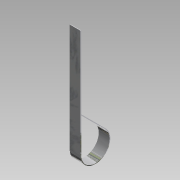
# Autodesk Inventor part: スタビライザ
Saved by Autodesk Inventor 2017 (Build 210142000, 142)
## iProperties
Part Number: スタビライザ
Material: アルミニウム
Document SubType Name: Modeling
Designer: HISAAKI
Density: 2.7 g/cm^3
Appearance: サテン
Author: HISAAKI
Autodesk Inventor part; units mm, degrees
ref_plane "YZ Plane" through (0, 0, 0) normal (1, 0, 0) x (0, 1, 0)
ref_plane "XZ Plane" through (0, 0, 0) normal (0, 1, 0) x (-1, 0, 0)
ref_plane "XY Plane" through (0, 0, 0) normal (0, 0, 1) x (1, 0, 0)
sketch "スケッチ3" plane through (0, 0, 0) normal (1, 0, 0) x (0, 1, 0)
  line L0 (0, 0) -> (0, -150)
  line L1 (0, 0) -> (0, -100)
  arc A0 (0, -150) -> (35.3553, -135.3553) centre (20.7107, -150) ccw
  line L2 (0, -150) -> (20.7107, -150) construction
  line L3 (35.3553, -135.3553) -> (20.7107, -150) construction
  line L4 (35.3553, -135.3553) -> (0, -100)
  line L5 (0, 0) -> (1, 0)
  arc A1 (1, -150) -> (34.6482, -136.0624) centre (20.7107, -150) ccw
  line L6 (34.6482, -136.0624) -> (1, -102.4142)
  line L7 (1, -150) -> (1, -102.4142)
  dimension "d13" = 150
  dimension "d14" = 100
  dimension "d16" = 135
  dimension "d17" = 1
  constraints: 16 end point, 4 point on circle, 3 point on line, 2 centre point, 2 tangent, 1 coincident, 1 horizontal, 1 parallel, 1 perpendicular, 1 vertical
  measures "d13" distance of L0.start L0.end
  measures "d14" distance of L0.start L1.end
  measures "d16" angle of L3 L2
  measures "d17" distance of L0.start L5.end
extrude "押し出し3" add sketch "スケッチ3" along normal blind 15
sketch "スケッチ4" plane through (0, 0, 0) normal (-1, 0, 0) x (0, 0, 1)
  line L0 (-100, 0) -> (-150, 0) projected
  line L1 (-100, 0) -> (0, 0)
  line L2 (0, 0) -> (0, 1)
  line L3 (0, 1) -> (-101, 1)
  line L4 (-135.3553, 35.3553) -> (-100, 0) projected
  line L5 (-101, 1) -> (-100, 0)
  dimension "d20" = 1
  constraints: 8 end point, 2 perpendicular, 1 collinear, 1 horizontal, 1 point on line
  measures "d20" distance of L1.end L2.end
extrude "押し出し4" add sketch "スケッチ4" against normal blind 15
sketch "スケッチ5" plane through (15, 0, 0) normal (1, 0, 0) x (0, 0, -1)
  line L0 (0, 0) -> (150, 0) projected
  line L1 (0, 0) -> (-10, 0)
  line L2 (-10, 0) -> (-10, 1)
  line L3 (-10, 1) -> (0, 1)
  line L4 (0, 1) -> (0, 0)
  dimension "d23" = 10
  dimension "d24" = 1
  constraints: 8 end point, 3 perpendicular, 1 horizontal
  measures "d23" distance of L0.start L1.end
  measures "d24" distance of L1.end L2.end
extrude "押し出し5" add sketch "スケッチ5" against normal blind 15
